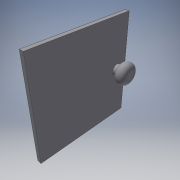
# Autodesk Inventor part: front door (for assembly)
Saved by Autodesk Inventor 2016 (Build 200138000, 138)
## iProperties
Created: 2017-10-23
Part Number: front door (for assembly)
Material: Generic
Document SubType Name: Modeling
Designer: student
Density: 1 g/cm^3
Appearance: Default
Author: student
Autodesk Inventor part; units mm, degrees
ref_plane "YZ Plane" through (0, 0, 0) normal (1, 0, 0) x (0, 1, 0)
ref_plane "XZ Plane" through (0, 0, 0) normal (0, 1, 0) x (-1, 0, 0)
ref_plane "XY Plane" through (0, 0, 0) normal (0, 0, 1) x (1, 0, 0)
sketch "Sketch1" plane through (0, 0, 0) normal (1, 0, 0) x (0, 1, 0)
  line L0 (-228.6, 228.6) -> (228.6, 228.6)
  line L1 (228.6, 228.6) -> (228.6, -228.6)
  line L2 (228.6, -228.6) -> (-228.6, -228.6)
  line L3 (-228.6, -228.6) -> (-228.6, 228.6)
  line L4 (-228.6, 228.6) -> (228.6, -228.6) construction
  line L5 (228.6, 228.6) -> (-228.6, -228.6) construction
  point P0 (0, 0)
  dimension "d0" = 457.2
  dimension "d1" = 457.2
  constraints: 12 end point, 2 midpoint, 2 parallel, 1 horizontal, 1 perpendicular
  measures "d0" distance of L1.end L2.end
  measures "d1" distance of L0.end L1.end
extrude "Extrusion1" add sketch "Sketch1" along normal blind 19.05
sketch "Sketch2" plane through (19.05, 0, 0) normal (1, 0, 0) x (0, 0, -1)
  circle A0 centre (177.8, 0) radius 25.4
  line L0 (228.6, -228.6) -> (228.6, 228.6) projected
  point P0 (0, 0)
  point P1 (228.6, 0)
  dimension "d4" = 50.8
  dimension "d5" = 50.8
  constraints: 1 centre point, 1 horizontal alignment, 1 midpoint
  measures "d4" diameter of A0
  measures "d5" distance from line of L0 A0.centre
extrude "Extrusion2" add sketch "Sketch2" along normal blind 19.05
sketch "Sketch3" plane through (38.1, 0, -177.8) normal (1, 0, 0) x (0, 0, -1)
  circle A0 centre (0, 0) radius 50.8
  line L0 (50.8, -228.6) -> (50.8, 228.6) projected
  point P0 (-177.8, 0)
  dimension "d8" = 50.8
  dimension "d9" = 101.6
  constraints: 1 centre point
  measures "d8" distance from line of L0 A0.centre
  measures "d9" diameter of A0
extrude "Extrusion3" add sketch "Sketch3" along normal blind 50.8
fillet "Fillet1" radius 25.4 2 edges at (88.9, 0, -127) (38.1, 0, -127)
body "Solid1"
